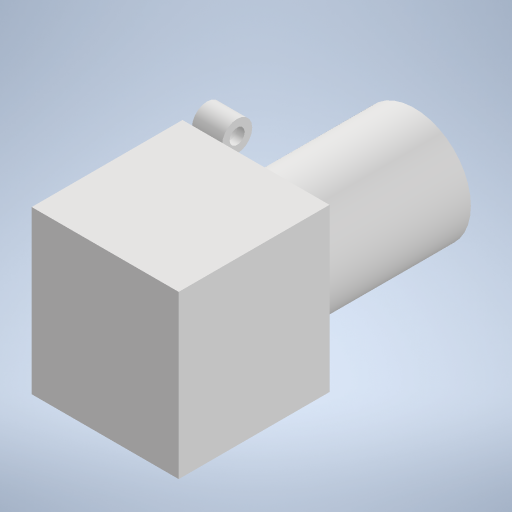
# Autodesk Inventor part: Pump
Saved by Autodesk Inventor 2024.2 (Build 282272000, 272)
## iProperties
Created: 2024-03-11
Part Number: Pump
Material: Ogólny
Document SubType Name: Modeling
Designer: Daniel
Density: 1 g/cm^3
Appearance: Domyślna
Author: Daniel
Autodesk Inventor part; units mm, degrees
ref_plane "YZ Plane" through (0, 0, 0) normal (1, 0, 0) x (0, 1, 0)
ref_plane "XZ Plane" through (0, 0, 0) normal (0, 1, 0) x (-1, 0, 0)
ref_plane "XY Plane" through (0, 0, 0) normal (0, 0, 1) x (1, 0, 0)
sketch "Szkic1" plane through (0, 0, 0) normal (0, 0, 1) x (1, 0, 0)
  circle A0 centre (0, 0) radius 15
  dimension "d0" = 30
  constraints: 1 centre point, 1 coincident
  measures "d0" diameter of A0
extrude "Wyciągnięcie proste1" add sketch "Szkic1" along normal blind 40
sketch "Szkic2" plane through (0, 0, 40) normal (0, 0, 1) x (1, 0, 0)
  line L0 (-17.5, 21.5) -> (17.5, 21.5)
  line L1 (17.5, 21.5) -> (17.5, -21.5)
  line L2 (17.5, -21.5) -> (-17.5, -21.5)
  line L3 (-17.5, -21.5) -> (-17.5, 21.5)
  line L4 (-17.5, 21.5) -> (17.5, -21.5) construction
  line L5 (17.5, 21.5) -> (-17.5, -21.5) construction
  point P0 (0, 0)
  dimension "d3" = 35
  dimension "d4" = 43
  constraints: 12 end point, 2 midpoint, 2 parallel, 1 horizontal, 1 perpendicular
  measures "d3" distance of L1.end L2.end
  measures "d4" distance of L0.end L1.end
extrude "Wyciągnięcie proste2" add sketch "Szkic2" along normal blind 40
sketch "Szkic3" plane through (0, 0, 40) normal (0, 0, -1) x (-1, 0, 0)
  circle A0 centre (0, 0) radius 15 projected
  line L0 (15, 0) -> (15, 20)
  circle A1 centre (0, 0) radius 15 projected
  line L1 (15, 20) -> (12, 20)
  line L2 (12, 20) -> (12, 9)
  dimension "d7" = 20
  dimension "d8" = 3
  constraints: 6 end point, 2 vertical, 1 horizontal, 1 point on circle, 1 tangent, 2 other
  measures "d7" distance of L0.start L0.end
  measures "d8" distance of L0.end L1.end
extrude "Wyciągnięcie proste3" add sketch "Szkic3" along normal blind 5 contours A0 L2 L1 L0
sketch "Szkic4" plane through (-12, 9, 40) normal (1, 0, 0) x (0, 0, -1)
  circle A0 centre (5, 11) radius 4
  point P0 (40, -9)
  dimension "d11" = 8
  constraints: 1 centre point, 1 coincident
  measures "d11" diameter of A0
extrude "Wyciągnięcie proste4" add sketch "Szkic4" against normal blind 8
sketch "Szkic5" plane through (-20, 20, 35) normal (-1, 0, 0) x (0, 0, 1)
  circle A0 centre (0, 0) radius 4 projected
  circle A1 centre (0, 0) radius 3
  circle A2 centre (0, 0) radius 2
  point P0 (-35, -20)
  dimension "d14" = 6
  dimension "d17" = 4
  constraints: 2 centre point, 2 coincident
  measures "d14" diameter of A1
  measures "d17" diameter of A2
extrude "Wyciągnięcie proste5" cut sketch "Szkic5" against normal blind 6 contours A1 | A2
extrude "Wyciągnięcie proste6" cut sketch "Szkic5" against normal through all contours A2
mirror "Odbij1" about plane through (0, 0, 0) normal (0, 1, 0) of "Wyciągnięcie proste6", "Wyciągnięcie proste5", "Wyciągnięcie proste4", "Wyciągnięcie proste3"
move faces "Przesuń1" translate (-4, 0, 0) faces at (-17.5, 7.1667, 53.3333)
